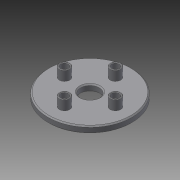
# Autodesk Inventor part: Gear_Base_11.4mmD_4x_4.7mmW_3mmH_4.4mmE
Saved by Autodesk Inventor 2015 (Build 190159000, 159)
## iProperties
Created: 2014-08-10
Part Number: Gear_Base_11.4mmD_4x_4.7mmW_3mmH_4.4mmE
Material: Generic
Document SubType Name: Modeling
Designer: User
Density: 1 g/cm^3
Appearance: Default
Author: User
Autodesk Inventor part; units mm, degrees
ref_plane "YZ Plane" through (0, 0, 0) normal (1, 0, 0) x (0, 1, 0)
ref_plane "XZ Plane" through (0, 0, 0) normal (0, 1, 0) x (-1, 0, 0)
ref_plane "XY Plane" through (0, 0, 0) normal (0, 0, 1) x (1, 0, 0)
sketch "Sketch1" plane through (0, 0, 0) normal (0, 0, 1) x (1, 0, 0)
  circle A0 centre (0, 0) radius 18.8
  circle A1 centre (0, 0) radius 4.15
  circle A2 centre (11.4, 0) radius 1.7
  circle A3 centre (0, 11.4) radius 1.7
  circle A4 centre (-11.4, 0) radius 1.7
  circle A5 centre (0, -11.4) radius 1.7
  dimension "d2" = 37.6
  dimension "d3" = 8.3
  dimension "d6" = 3.4
  dimension "d7" = 11.4
  dimension "d10" = 360
  constraints: 6 centre point, 2 coincident, 1 horizontal alignment, 9 other
  measures "d2" diameter of A0
  measures "d3" diameter of A1
  measures "d6" diameter of A2
  measures "d7" distance of point (0, 0) A2.centre
extrude "Extrusion1" add sketch "Sketch1" along normal blind 3
sketch "Sketch2" plane through (0, 0, 3) normal (0, 0, 1) x (1, 0, 0)
  circle A0 centre (0, 0) radius 4.15 projected
  circle A1 centre (0, -11.4) radius 1.7 projected
  circle A2 centre (-11.4, 0) radius 1.7 projected
  circle A3 centre (0, 11.4) radius 1.7 projected
  circle A4 centre (11.4, 0) radius 1.7 projected
  circle A5 centre (0, 0) radius 18.8 projected
  circle A6 centre (11.4, 0) radius 2.35
  circle A7 centre (0, 11.4) radius 2.35
  circle A8 centre (-11.4, 0) radius 2.35
  circle A9 centre (0, -11.4) radius 2.35
  dimension "d12" = 4.7
  dimension "d15" = 360
  constraints: 4 centre point, 1 coincident, 9 other
  measures "d12" diameter of A6
extrude "Extrusion2" add sketch "Sketch2" along normal blind 4.4 contours A6 | A7 | A8 | A9
chamfer "Chamfer1" distance 0.5 angle 45 8 edges at (-18.8, 0, 3) (-18.8, 0, 0) (-4.15, 0, 3) (-4.15, 0, 0) (-1.7, -11.4, 0) (9.7, 0, 0) (-1.7, 11.4, 0) (-13.1, 0, 0)
chamfer "Chamfer2" distance 0.2 angle 45 8 edges at (-13.75, 0, 7.4) (-13.1, 0, 7.4) (-1.7, 11.4, 7.4) (-2.35, 11.4, 7.4) (9.7, 0, 7.4) (9.05, 0, 7.4) (-1.7, -11.4, 7.4) (-2.35, -11.4, 7.4)
body "Solid1"
